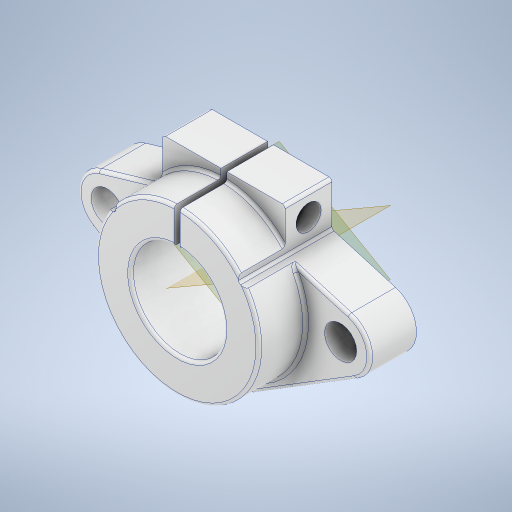
# Autodesk Inventor part: SHF16
Saved by Autodesk Inventor 2024 (Build 280153000, 153)
## iProperties
Created: 2024-12-28
Part Number: SHF16
Material: Aluminum 6061
Document SubType Name: Modeling
Designer: Ishaan
Density: 2.7 g/cm^3
Appearance: Aluminum - Flat
Author: Ishaan
Autodesk Inventor part; units mm, degrees
ref_plane "YZ Plane" through (0, 0, 0) normal (1, 0, 0) x (0, 1, 0)
ref_plane "XZ Plane" through (0, 0, 0) normal (0, 1, 0) x (-1, 0, 0)
sketch "Sketch1" plane through (0, 0, 0) normal (0, 0, 1) x (1, 0, 0)
  circle A0 centre (0, 0) radius 14
  circle A1 centre (0, 0) radius 8
  line L0 (-20, 0) -> (20, 0) construction
  line L1 (25, -15.5) -> (-25, -15.5) construction
  line L2 (-25, -15.5) -> (-25, 15.5) construction
  line L3 (-25, 15.5) -> (25, 15.5) construction
  line L4 (25, 15.5) -> (25, -15.5) construction
  line L5 (25, -15.5) -> (-25, 15.5) construction
  line L6 (-25, -15.5) -> (25, 15.5) construction
  line L7 (20, 0) -> (-20, 0) construction
  line L8 (20, 5) -> (-20, 5)
  line L9 (-20, -5) -> (20, -5)
  arc A2 (20, -5) -> (20, 5) centre (20, 0) ccw
  arc A3 (-20, 5) -> (-20, -5) centre (-20, 0) ccw
  circle A4 centre (0, 0) radius 15.5 construction
  line L10 (-22.625, -4.2555) -> (-4.396, -15.5)
  line L11 (-4.396, -15.5) -> (4.396, -15.5)
  line L12 (4.396, -15.5) -> (22.625, -4.2555)
  line L13 (10.5, 15.5) -> (-10.5, 15.5)
  line L14 (-10.5, 15.5) -> (-10.5, 8)
  line L15 (-10.5, 8) -> (10.5, 8)
  line L16 (10.5, 8) -> (10.5, 15.5)
  line L17 (10.5, 15.5) -> (-10.5, 8) construction
  line L18 (-10.5, 15.5) -> (10.5, 8) construction
  line L19 (-21.4084, 4.7975) -> (-10.5, 8)
  line L20 (10.5, 8) -> (21.4084, 4.7975)
  line L21 (-10.5, 11.75) -> (10.5, 11.75) construction
  point P0 (0, 11.75)
  point P1 (0, 15.5)
  point P2 (11.7329, 7.6381)
  point P3 (10.5, 9.2601)
  point P4 (-10.5, 9.2601)
  point P5 (-11.7329, 7.6381)
  dimension "d0" = 28
  dimension "d1" = 16
  dimension "d2" = 40
  dimension "d3" = 50
  dimension "d4" = 31
  dimension "d5" = 7.5
  dimension "d6" = 21
  constraints: 46 end point, 12 tangent, 9 midpoint, 8 point on circle, 6 coincident, 6 equal length, 5 centre point, 3 horizontal, 2 perpendicular, 2 point on line, 2 vertical alignment, 1 collinear
  measures "d0" diameter of A0
  measures "d1" diameter of A1
  measures "d2" distance of L0.start L0.end
  measures "d3" distance of L2.end L3.end
  measures "d4" distance of L1.end L2.end
  measures "d5" distance of L14.end L13.end
  measures "d6" distance of L14.end L15.end
extrude "Extrusion1" add sketch "Sketch1" along normal blind 8 contours A0 L9 A1 L8 | A0 L8 A2 L9 | L8 A1 L15 L20 A0 | A0 L20 A2 L8 | L9 A2 L12 L11 L10 A3 A0 | A0 L9 A1 | L9 A3 L8 A0 | A0 L8 A1 L9 | L16 L15 L14 A0 | A0 L14 L13 L16 | A1 L8 A0 L19 L15 | L8 A3 L19 A0
extrude "Extrusion2" add sketch "Sketch1" along normal blind 16 contours A0 L9 A1 L8 | L8 A1 L15 L20 A0 | A0 L9 A1 | A0 L8 A1 L9 | L16 L15 L14 A0 | A1 L8 A0 L19 L15
fillet "Fillet1" radius 2 2 edges at (-4.396, -15.5, 4) (4.396, -15.5, 4)
fillet "Fillet4" radius 0.5 9 edges at (24.9555, 0.6659, 8) (13.7519, -9.7289, 8) (4.3745, -15.4241, 8) (0, -15.5, 8) (-4.3745, -15.4241, 8) (-13.7519, -9.7289, 8) (-24.9555, 0.6659, 8) (-16.5707, 6.2178, 8) (16.5707, 6.2178, 8)
fillet "Fillet2" radius 0.5 4 edges at (0, -14, 16) (0, 14, 16) (0, -14, 8) (0, 14, 8)
fillet "Fillet3" radius 0.5 2 edges at (10.5, 8, 8) (-10.5, 8, 8)
fillet "Fillet5" radius 0.5 2 edges at (-8, 0, 16) (-8, 0, 0)
fillet "Fillet6" radius 0.5 2 edges at (10.5, 15.5, 4) (-10.5, 15.5, 4)
hole "Hole1" at (20, 0, 0) at (-20, 0, 0) direction (0, 0, 1) diameter 5.5 end through all
ref_plane "Work Plane1" through (0, 0, 4) normal (0, 0, 1) x (1, 0, 0)
sketch "Sketch2" plane through (10.5, 9.2601, 15.5) normal (1, 0, 0) x (0, 0, -1)
  line L0 (11.5, -30.9601) -> (11.5, 12.4399) construction
  point P0 (15.5, -9.2601)
  point P1 (15.5, 2.4899)
  point P2 (15.5, 2.4899)
  point P3 (15.5, 2.4899)
  point P4 (11.5, 2.4899)
  constraints: 1 horizontal alignment, 1 point on line
hole "Hole2" at (10.5, 11.75, 4) direction (-1, 0, 0) diameter 3.242 end through all counterbore diameter 4.3 counterbore depth 10.5 thread size "M4x0.7" class "6H" standard "ANSI Metric M Profile"
sketch "Sketch3" plane through (0, 0, 16) normal (0, 0, 1) x (1, 0, 0)
  circle A0 centre (0, 0) radius 8 projected
  line L0 (0.5, 15.5) -> (-0.5, 15.5)
  line L1 (-0.5, 15.5) -> (-0.5, -15.5)
  line L2 (-0.5, -15.5) -> (0.5, -15.5)
  line L3 (0.5, -15.5) -> (0.5, 15.5)
  line L4 (0.5, 15.5) -> (-0.5, -15.5) construction
  line L5 (-0.5, 15.5) -> (0.5, -15.5) construction
  line L6 (10, 15.5) -> (-10, 15.5) projected
  point P0 (0.5, -7.9844)
  point P1 (-0.5, -7.9844)
  dimension "d31" = 1
  constraints: 12 end point, 2 midpoint, 2 parallel, 1 collinear, 1 horizontal, 1 perpendicular
  measures "d31" distance of L2.end L1.end
extrude "Extrusion3" cut sketch "Sketch3" against normal up to surface (16 mm away) contours L3 A0 L1 | A0 L1 L0 L3
sketch "Sketch4" plane through (0, 0, 0) normal (0, 0, 1) x (1, 0, 0)
  line L0 (29.4856, 6.0705) -> (-9.4856, 28.5705) construction
  line L1 (-9.4856, 28.5705) -> (-29.4856, -6.0705) construction
  line L2 (-29.4856, -6.0705) -> (9.4856, -28.5705) construction
  line L3 (9.4856, -28.5705) -> (29.4856, 6.0705) construction
  line L4 (29.4856, 6.0705) -> (-29.4856, -6.0705) construction
  line L5 (-9.4856, 28.5705) -> (9.4856, -28.5705) construction
  line L6 (24.4856, -2.5897) -> (-14.4856, 19.9103) construction
  line L7 (-14.4856, 19.9103) -> (-24.4856, 2.5897) construction
  line L8 (-24.4856, 2.5897) -> (14.4856, -19.9103) construction
  line L9 (14.4856, -19.9103) -> (24.4856, -2.5897) construction
  line L10 (24.4856, -2.5897) -> (-24.4856, 2.5897) construction
  line L11 (-14.4856, 19.9103) -> (14.4856, -19.9103) construction
  circle A0 centre (-20, 0) radius 2.75 construction
  line L12 (24.4856, 2.5897) -> (-14.4856, -19.9103) construction
  line L13 (-14.4856, -19.9103) -> (-24.4856, -2.5897) construction
  line L14 (-24.4856, -2.5897) -> (14.4856, 19.9103) construction
  line L15 (14.4856, 19.9103) -> (24.4856, 2.5897) construction
  line L16 (24.4856, 2.5897) -> (-24.4856, -2.5897) construction
  line L17 (-14.4856, -19.9103) -> (14.4856, 19.9103) construction
  point P0 (0, 0)
  dimension "d34" = 40
  dimension "d35" = 20
  dimension "d36" = 45
  dimension "d37" = 20
  constraints: 36 end point, 6 midpoint, 6 parallel, 3 perpendicular, 2 point on line, 1 collinear, 1 equal length
  measures "d34" distance of L1.end L0.end
  measures "d35" distance of L7.end L6.end
  measures "d36" distance of L1.end L2.end
  measures "d37" distance of L12.end L13.end
ref_plane "Work Plane2" through (0, 0, 0) normal (-0.5, -0.866, 0) x (0.866, -0.5, 0)
ref_plane "Work Plane3" through (0, 0, 0) normal (-0.5, 0.866, 0) x (-0.866, -0.5, 0)
body "Solid1"
